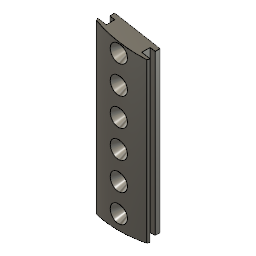
Sensor Rail Left v6 (Autodesk Fusion 360 design; units mm, degrees)
Autodesk Fusion 360 part; units mm, degrees
sketch "Sketch1" plane through (0, 0, 0) normal (0, 1, 0) x (1, 0, 0)
  line L0 (25, 18) -> (-25, 18) construction
  line L1 (-25, 18) -> (-25, -18) construction
  line L2 (-25, -18) -> (25, -18) construction
  line L3 (25, -18) -> (25, 18) construction
  line L4 (25, 18) -> (-25, -18) construction
  line L5 (-25, 18) -> (25, -18) construction
  arc A0 (25, 18) -> (-25, 18) centre (0, -84.666667) ccw
  arc A1 (-25, -18) -> (25, -18) centre (0, 84.666667) ccw
  arc A2 (25, -18) -> (25, 18) centre (-27.5, 0) ccw
  arc A3 (-25, 18) -> (-25, -18) centre (27.5, 0) ccw
  line L6 (-25.79165, -15.5) -> (-17.5, -15.5)
  line L7 (-17.5, -15.5) -> (-17.5, -7.2)
  line L8 (-17.5, -7.2) -> (-22.5, -7.2)
  line L9 (-22.5, -7.2) -> (-22.5, -2.2)
  line L10 (-22.5, -2.2) -> (22.5, -2.2)
  line L11 (22.5, -2.2) -> (22.5, -7.2)
  line L12 (22.5, -7.2) -> (17.5, -7.2)
  line L13 (17.5, -7.2) -> (17.5, -15.5)
  line L14 (17.5, -15.5) -> (25.79165, -15.5)
  dimension "d1" = 50
  dimension "d2" = 36
  dimension "d3" = 42
  dimension "d4" = 56
  dimension "d33" = 5.5
  dimension "d34" = 35
  dimension "d35" = 45
  dimension "d36" = 8.3
  dimension "d37" = 5
  measures "d33" distance of L6
  measures "d34" distance of L7 L13
extrude "Extrude1" add sketch "Sketch1" along normal blind 170 contours A1 A2 A3 L6 L7 L8 L9 L10 L11 L12 L13 L14 picked at (0, -11.8)
sketch "Sketch8" plane through (0, 0, 0) normal (0, 0, 1) x (1, 0, 0)
  line L0 (-28, 170) -> (28, 160)
  line L1 (25, 170) -> (-25, 170)
  line L2 (28, 160) -> (28, 175)
  line L3 (28, 175) -> (-28, 175)
  line L4 (-28, 175) -> (-28, 170)
  line L5 (31, 178) -> (-31, 178)
  line L6 (-31, 178) -> (-31, 167.488258)
  line L7 (-31, 167.488258) -> (31, 156.416829)
  line L8 (31, 156.416829) -> (31, 178)
  dimension "d38" = 160
  dimension "d39" = 170
  dimension "d40" = 3
extrude "Extrude7" cut sketch "Sketch8" along normal through all contours L0 L2 L3 L4 | L5 L6 L7 L8 picked at (9.333333, 168.333333) picked at (9.333333, 161.301696)
sketch "Sketch9" plane through (0, 0, 2.2) normal (0, 0, -1) x (-1, 0, 0)
  line L0 (22.5, 165.970401) -> (-22.5, 157.934687)
  line L1 (-22.5, 157.934687) -> (-22.5, 0)
  line L2 (-22.5, 0) -> (22.5, 0)
  line L3 (22.5, 0) -> (22.5, 165.970401)
  circle A0 centre (0, 14.5) radius 2.5
  dimension "d42" = 5
  dimension "d43" = 14.5
  measures "d42" diameter of A0
extrude "Extrude8" cut sketch "Sketch9" against normal through all contours A0 picked at (-1.150702, 14.363686)
chamfer "Chamfer1" distance 6 distance2 14 1 edges at (-2.5, 14.5, 20.970422) measured on face at (-15.924, 110.05648, 19.793233)
pattern_linear "R-Pattern1" count 6 spacing 27.5 along (0, 1, 0) of "Extrude8", "Chamfer1"
